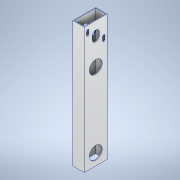
# Autodesk Inventor part: 2x1 Front with motor mount
Saved by Autodesk Inventor 2020 (Build 240168000, 168)
## iProperties
Created: 2020-01-27
Part Number: 2x1 Front with motor mount
Material: Aluminum 6061
Document SubType Name: Modeling
Designer: 1cikaychapman
Density: 2.7 g/cm^3
Appearance: Aluminum - Flat
Author: 1cikaychapman
Autodesk Inventor part; units mm, degrees
ref_plane "YZ Plane" through (0, 0, 0) normal (1, 0, 0) x (0, 1, 0)
ref_plane "XZ Plane" through (0, 0, 0) normal (0, 1, 0) x (-1, 0, 0)
ref_plane "XY Plane" through (0, 0, 0) normal (0, 0, 1) x (1, 0, 0)
sketch "Sketch1" plane through (0, 0, 0) normal (0, 1, 0) x (-1, 0, 0)
  line L0 (-12.7, 25.4) -> (12.7, 25.4)
  line L1 (12.7, 25.4) -> (12.7, -25.4)
  line L2 (12.7, -25.4) -> (-12.7, -25.4)
  line L3 (-12.7, -25.4) -> (-12.7, 25.4)
  line L4 (-12.7, 25.4) -> (12.7, -25.4) construction
  line L5 (12.7, 25.4) -> (-12.7, -25.4) construction
  line L6 (11.1125, 23.8125) -> (-11.1125, 23.8125)
  line L7 (-11.1125, 23.8125) -> (-11.1125, -23.8125)
  line L8 (-11.1125, -23.8125) -> (11.1125, -23.8125)
  line L9 (11.1125, -23.8125) -> (11.1125, 23.8125)
  line L10 (11.1125, 23.8125) -> (-11.1125, -23.8125) construction
  line L11 (-11.1125, 23.8125) -> (11.1125, -23.8125) construction
  point P0 (0, 0)
  dimension "d0" = 25.4
  dimension "d1" = 50.8
  dimension "d2" = 22.225
  dimension "d3" = 47.625
  constraints: 24 end point, 4 midpoint, 4 parallel, 2 horizontal, 2 perpendicular
  measures "d0" distance of L1.end L2.end
  measures "d1" distance of L0.end L1.end
  measures "d2" distance of L8.end L7.end
  measures "d3" distance of L7.end L6.end
extrude "Extrusion1" add sketch "Sketch1" along normal blind 279.4
sketch "Sketch2" plane through (12.7, 0, 25.4) normal (1, 0, 0) x (0, 0, -1)
  line L0 (0, 279.4) -> (50.8, 279.4) projected
  line L1 (0, 0) -> (0, 279.4) projected
  point P0 (25.4, 0)
  point P1 (25.4, 190.5)
  dimension "d21" = 25.4
  dimension "d24" = 190.5
  measures "d21" distance from line of L1 point (25.4, 190.5)
  measures "d24" distance of point (25.4, 0) point (25.4, 190.5)
hole "Hole1" at (12.7, 190.5, 0) direction (-1, 0, 0) diameter 28.575 end through all
sketch "Sketch3" plane through (12.7, 0, 25.4) normal (1, 0, 0) x (0, 0, -1)
  line L0 (50.8, 0) -> (50.8, 279.4) projected
  line L1 (0, 0) -> (50.8, 0) projected
  point P0 (25.4, 0)
  point P1 (25.4, 25.4)
  dimension "d22" = 25.4
  dimension "d23" = 25.4
  measures "d22" distance from line of L0 point (25.4, 25.4)
  measures "d23" distance from line of L1 point (25.4, 25.4)
hole "Hole2" at (12.7, 25.4, 0) direction (-1, 0, 0) diameter 28.575 end through all
sketch "Sketch5" plane through (12.7, 0, 25.4) normal (1, 0, 0) x (0, 0, -1)
  line L0 (25.4, 254) -> (25.4, 246.38) construction
  line L1 (17.78, 254) -> (17.78, 246.38)
  line L2 (33.02, 246.38) -> (33.02, 254)
  arc A0 (33.02, 254) -> (17.78, 254) centre (25.4, 254) ccw
  arc A1 (17.78, 246.38) -> (33.02, 246.38) centre (25.4, 246.38) ccw
  line L3 (0, 279.4) -> (50.8, 279.4) projected
  point P0 (25.4, 0)
  point P1 (25.4, 250.19)
  dimension "d34" = 7.62
  dimension "d35" = 15.24
  dimension "d36" = 25.4
  constraints: 8 end point, 4 point on circle, 4 tangent, 2 centre point, 1 midpoint, 1 parallel, 1 vertical
  measures "d34" distance of L0.start L0.end
  measures "d35" diameter of A1
  measures "d36" distance from line of L3 L0.start
extrude "Extrusion2" cut sketch "Sketch5" against normal through all
sketch "Sketch6" plane through (12.7, 0, 25.4) normal (1, 0, 0) x (0, 0, -1)
  line L0 (7.5819, 268.7054) -> (43.2181, 268.7054) construction
  line L1 (43.2181, 268.7054) -> (43.2181, 233.0692) construction
  line L2 (43.2181, 233.0692) -> (7.5819, 233.0692) construction
  line L3 (7.5819, 233.0692) -> (7.5819, 268.7054) construction
  line L4 (7.5819, 268.7054) -> (43.2181, 233.0692) construction
  line L5 (43.2181, 268.7054) -> (7.5819, 233.0692) construction
  line L6 (7.5819, 268.7054) -> (7.5819, 261.0854) construction
  line L7 (4.8514, 268.7054) -> (4.8514, 261.0854)
  line L8 (10.3124, 261.0854) -> (10.3124, 268.7054)
  arc A0 (10.3124, 268.7054) -> (4.8514, 268.7054) centre (7.5819, 268.7054) ccw
  arc A1 (4.8514, 261.0854) -> (10.3124, 261.0854) centre (7.5819, 261.0854) ccw
  line L9 (43.2181, 233.0692) -> (43.2181, 240.6892) construction
  line L10 (45.9486, 233.0692) -> (45.9486, 240.6892)
  line L11 (40.4876, 240.6892) -> (40.4876, 233.0692)
  arc A2 (40.4876, 233.0692) -> (45.9486, 233.0692) centre (43.2181, 233.0692) ccw
  arc A3 (45.9486, 240.6892) -> (40.4876, 240.6892) centre (43.2181, 240.6892) ccw
  point P0 (25.4, 0)
  point P1 (25.4, 250.8873)
  point P2 (7.5819, 264.8954)
  point P3 (43.2181, 236.8792)
  dimension "d39" = 35.6362
  dimension "d40" = 35.6362
  dimension "d46" = 7.62
  dimension "d47" = 5.461
  dimension "d48" = 7.62
  dimension "d49" = 5.461
  constraints: 28 end point, 8 point on circle, 8 tangent, 4 centre point, 4 midpoint, 4 parallel, 2 point on line, 1 coincident, 1 horizontal, 1 perpendicular
  measures "d39" distance of L1.end L2.end
  measures "d40" distance of L0.end L1.end
  measures "d46" distance of L6.start L6.end
  measures "d47" diameter of A1
  measures "d48" distance of L1.end L9.end
  measures "d49" diameter of A3
extrude "Extrusion3" cut sketch "Sketch6" against normal through all
sketch "Sketch7" plane through (-12.7, 0, -25.4) normal (-1, 0, 0) x (0, 0, 1)
  arc A0 (10.3124, 240.6892) -> (4.8514, 240.6892) centre (7.5819, 240.6892) ccw projected
  line L0 (7.5819, 240.6892) -> (7.5819, 232.5183) construction
  line L1 (3.1369, 240.6892) -> (3.1369, 232.5183)
  line L2 (12.0269, 232.5183) -> (12.0269, 240.6892)
  arc A1 (12.0269, 240.6892) -> (3.1369, 240.6892) centre (7.5819, 240.6892) ccw
  arc A2 (3.1369, 232.5183) -> (12.0269, 232.5183) centre (7.5819, 232.5183) ccw
  arc A3 (45.9486, 268.7054) -> (40.4876, 268.7054) centre (43.2181, 268.7054) ccw projected
  arc A4 (40.4876, 261.0854) -> (45.9486, 261.0854) centre (43.2181, 261.0854) ccw projected
  line L3 (43.2181, 268.7054) -> (43.2181, 261.0854) construction
  line L4 (38.7731, 268.7054) -> (38.7731, 261.0854)
  line L5 (47.6631, 261.0854) -> (47.6631, 268.7054)
  arc A5 (47.6631, 268.7054) -> (38.7731, 268.7054) centre (43.2181, 268.7054) ccw
  arc A6 (38.7731, 261.0854) -> (47.6631, 261.0854) centre (43.2181, 261.0854) ccw
  point P0 (25.4, 0)
  point P1 (7.5819, 236.6038)
  point P2 (43.2181, 264.8954)
  dimension "d50" = 8.89
  dimension "d51" = 8.89
  constraints: 16 end point, 8 point on circle, 8 tangent, 4 centre point, 2 midpoint, 2 parallel, 2 vertical
  measures "d50" diameter of A2
  measures "d51" diameter of A6
extrude "Extrusion4" cut sketch "Sketch7" against normal blind 12.7
body "Solid1"
